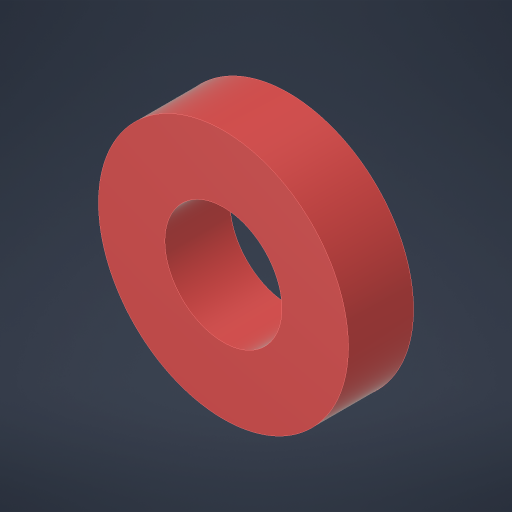
# Autodesk Inventor part: AR-018
Saved by Autodesk Inventor 2023.4 (Build 274418000, 418)
## iProperties
Created: 2025-02-15
Part Number: AR-018
Material: PC/ABS Plastic
Document SubType Name: Modeling
Designer: brand
Density: 0.357273 g/cm^3
Appearance: Smooth - Red
Author: brand
Autodesk Inventor part; units mm, degrees
ref_plane "YZ Plane" through (0, 0, 0) normal (1, 0, 0) x (0, 1, 0)
ref_plane "XZ Plane" through (0, 0, 0) normal (0, 1, 0) x (-1, 0, 0)
ref_plane "XY Plane" through (0, 0, 0) normal (0, 0, 1) x (1, 0, 0)
sketch "Sketch1" plane through (0, 0, 0) normal (0, 0, 1) x (1, 0, 0)
  circle A0 centre (0, 0) radius 11.176
  circle A1 centre (0, 0) radius 23.876
  dimension "d0" = 12.7
  dimension "d3" = 22.352
  constraints: 2 centre point, 2 coincident
  measures "d0" radial gap between concentric circles of A1 A0
  measures "d3" diameter of A0
extrude "Extrusion1" add sketch "Sketch1" along normal blind 12.446
body "Solid1"
